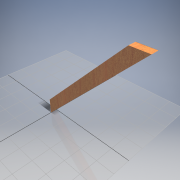
# Autodesk Inventor part: Back Angle Piece
Saved by Autodesk Inventor 2018 (Build 220112000, 112)
## iProperties
Created: 2016-08-30
Part Number: Back Angle Piece
Material: Wood
Document SubType Name: Modeling
Designer: jjsch
Density: 0.570257 g/cm^3
Appearance: Yellow Pine - Solid Natural Low Gloss
Mass: 1005.74 g
Surface Area: 1554.67 cm^2
Volume: 1763.66 cm^3
Author: jjsch
Autodesk Inventor part; units mm, degrees
ref_plane "YZ Plane" through (0, 0, 0) normal (1, 0, 0) x (0, 1, 0)
ref_plane "XZ Plane" through (0, 0, 0) normal (0, 1, 0) x (-1, 0, 0)
ref_plane "XY Plane" through (0, 0, 0) normal (0, 0, 1) x (1, 0, 0)
sketch "Sketch1" plane through (0, 0, 0) normal (0, 0, 1) x (1, 0, 0)
  line L0 (0, 0) -> (565.15, 565.15)
  line L1 (0, 88.9) -> (476.25, 565.15)
  line L2 (476.25, 565.15) -> (565.15, 565.15)
  line L3 (0, 0) -> (0, 88.9)
  dimension "d5" = 565.15
  dimension "d6" = 88.9
  dimension "d7" = 45
  constraints: 8 end point, 1 horizontal, 1 parallel, 1 perpendicular
  measures "d5" horizontal distance of L0.end L1.start
  measures "d6" distance of L1.start L0.start
  measures "d7" angle of L2 L0
extrude "Extrusion1" add sketch "Sketch1" along normal blind 38.1
body "Solid1"
